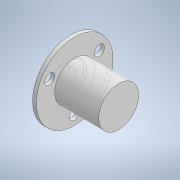
# Autodesk Inventor part: SRM-12-06A
Saved by Autodesk Inventor 2022 (Build 260153070, 153G)
## iProperties
Created: 2021-10-27
Part Number: SRM-12-06A
Material: Generic
Document SubType Name: Modeling
Designer: a laptop
Density: 1 g/cm^3
Appearance: Default
Author: a laptop
Autodesk Inventor part; units mm, degrees
ref_plane "YZ Plane" through (0, 0, 0) normal (1, 0, 0) x (0, 1, 0)
ref_plane "XZ Plane" through (0, 0, 0) normal (0, 1, 0) x (-1, 0, 0)
ref_plane "XY Plane" through (0, 0, 0) normal (0, 0, 1) x (1, 0, 0)
sketch "Sketch1" plane through (0, 0, 0) normal (0, 0, 1) x (1, 0, 0)
  line L0 (2.7, -6.25) -> (16.5, -6.25)
  line L1 (16.5, -6.25) -> (16.5, 0)
  line L2 (16.5, 0) -> (0, 0)
  line L3 (0, 0) -> (0, -2.5)
  line L4 (0, -2.5) -> (1.5, -2.5)
  line L5 (1.5, -2.5) -> (1.5, -12)
  line L6 (1.5, -12) -> (2.7, -12)
  line L7 (2.7, -12) -> (2.7, -6.25)
  dimension "d0" = 6.25
  dimension "d1" = 15
  dimension "d2" = 1.2
  dimension "d3" = 12
  dimension "d4" = 2.5
  dimension "d5" = 1.5
  constraints: 16 end point, 7 perpendicular, 1 coincident, 1 horizontal
  measures "d0" distance of L0.end L1.end
  measures "d1" horizontal distance of L0.end L5.end
  measures "d2" distance of L5.end L6.end
  measures "d3" distance from line of L2 L5.end
  measures "d4" distance of L2.end L3.end
  measures "d5" distance from line of L5 L3.end
revolve "Revolution1" add sketch "Sketch1" angle 360 about axis through (16.5, 0, 0) along (-1, 0, 0)
sketch "Sketch2" plane through (1.5, 0, 0) normal (-1, 0, 0) x (0, 0, 1)
  circle A0 centre (0, 0) radius 9 construction
  circle A1 centre (0, -9) radius 1.6
  line L0 (0, -16.8) -> (0, 16.8) projected
  circle A2 centre (7.7942, 4.5) radius 1.6
  circle A3 centre (-7.7942, 4.5) radius 1.6
  dimension "d7" = 18
  dimension "d8" = 3.2
  dimension "d11" = 360
  constraints: 3 centre point, 1 coincident, 1 point on line, 1 vertical alignment, 9 other
  measures "d8" diameter of A1
extrude "Extrusion1" cut sketch "Sketch2" against normal blind 1.2
sketch "Sketch3" plane through (0, 0, 0) normal (-1, 0, 0) x (0, 0, 1)
  circle A0 centre (0, 0) radius 2.5 projected
  point P0 (0, 0)
extrude "Extrusion2" add sketch "Sketch3" along normal blind 1.5
sketch "Sketch4" plane through (1.5, 0, 0) normal (-1, 0, 0) x (0, 0, 1)
  circle A0 centre (0, 0) radius 5
  dimension "d17" = 10
  constraints: 1 centre point, 1 coincident
  measures "d17" diameter of A0
extrude "Extrusion3" add sketch "Sketch4" along normal blind 1
body "Solid1"
